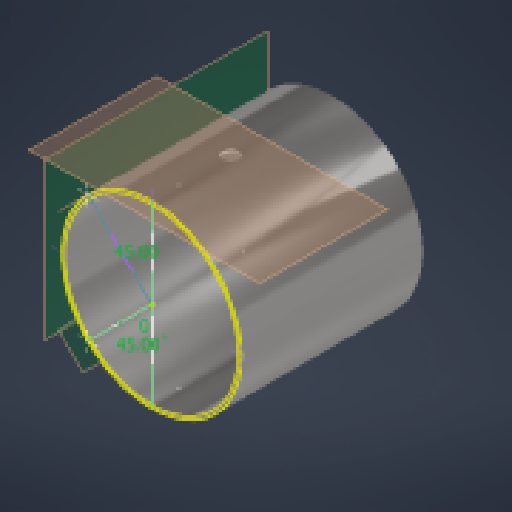
# Autodesk Inventor part: Electromagnetic cover body
Saved by Autodesk Inventor 2026.3 (Build 303398000, 398)
## iProperties
Created: 2026-08-03
Part Number: Electromagnetic cover body
Material: Generic
Document SubType Name: Sheet Metal
Designer: matot
Density: 1 g/cm^3
Sheet Metal Rule: Default_mm
Appearance: Default
Author: matot
Autodesk Inventor part; units mm, degrees
ref_plane "YZ Plane" through (0, 0, 0) normal (1, 0, 0) x (0, 1, 0)
ref_plane "XZ Plane" through (0, 0, 0) normal (0, 1, 0) x (-1, 0, 0)
ref_plane "XY Plane" through (0, 0, 0) normal (0, 0, 1) x (1, 0, 0)
sketch "Sketch1" plane through (0, 0, 0) normal (0, 0, 1) x (1, 0, 0)
  circle A0 centre (0, 0) radius 57
  circle A1 centre (0, 0) radius 55
  dimension "d0" = 114
  dimension "d1" = 110
  constraints: 2 centre point, 2 coincident
  measures "d0" diameter of A0
  measures "d1" diameter of A1
extrude "Extrusion1" add sketch "Sketch1" along normal blind 115
sketch "Sketch2" plane through (0, 0, 115) normal (0, 0, 1) x (1, 0, 0)
  circle A0 centre (0, 0) radius 57 projected
  point P0 (0, 57)
  constraints: 1 vertical alignment, 1 other
ref_plane "Work Plane1" through (0, 57, 115) normal (0, 1, 0) x (-1, 0, 0)
sketch "Sketch3" plane through (0, 57, 115) normal (0, 1, 0) x (-1, 0, 0)
  line L0 (57, 0) -> (-57, 0) projected
  point P0 (0, -115)
  point P1 (0, -50)
  dimension "d4" = 50
  measures "d4" distance from line of L0 point (0, -50)
hole "Hole1" at (0, 57, 65) direction (0, -1, 0) diameter 10 depth 20 tip angle 118
sketch "Sketch4" plane through (0, 0, 115) normal (0, 0, 1) x (1, 0, 0)
  circle A0 centre (0, 0) radius 57 projected
  point P0 (-57, 0)
  point P1 (57, 0)
  constraints: 1 horizontal alignment, 1 other
ref_plane "Work Plane3" through (-57, 0, 115) normal (-1, 0, 0) x (0, -1, 0)
sketch "Sketch6" plane through (0, 0, 115) normal (0, 0, 1) x (1, 0, 0)
  circle A0 centre (0, 0) radius 57 projected
  point P0 (0, 57)
  constraints: 1 vertical alignment, 1 other
ref_plane "Work Plane4" through (0, 57, 115) normal (0, 1, 0) x (-1, 0, 0)
sketch "Sketch7" plane through (0, 57, 115) normal (0, 1, 0) x (-1, 0, 0)
  line L0 (57, 0) -> (-57, 0) projected
  point P0 (0, -115)
  point P1 (0, -17.607)
  dimension "d20" = 17.607
  measures "d20" distance from line of point (0, -17.607) L0
hole "Hole3" at (0, 57, 97.393) direction (0, -1, 0) diameter 2 end through all
sketch "Sketch8" plane through (0, 0, 115) normal (0, 0, 1) x (1, 0, 0)
  circle A0 centre (0, 0) radius 57 projected
  circle A1 centre (0, 0) radius 55 projected
  line L0 (-40.3051, -40.3051) -> (0, 0)
  line L1 (0, -57) -> (0, 0)
  line L2 (-40.3051, 40.3051) -> (0, -0.029)
  line L3 (0, -0.029) -> (0, 57)
  dimension "d28" = 45
  dimension "d29" = 45
  dimension "d30" = 0
  constraints: 8 end point, 4 point on circle, 2 vertical
  measures "d30" horizontal distance of point (0, 0) L2.end
ref_plane "Work Plane5" through (-40.3051, -40.3051, 115) normal (-0.7071068, -0.7071068, 0) x (0.7071068, -0.7071068, 0)
ref_plane "Work Plane6" through (-40.3051, 40.3051, 115) normal (-0.7071068, 0.7071068, 0) x (-0.7071068, -0.7071068, 0)
sketch "Sketch9" plane through (-40.3051, 40.3051, 115) normal (-0.7071068, 0.7071068, 0) x (-0.7071068, -0.7071068, 0)
  line L0 (57, 0) -> (-57, 0) projected
  point P0 (0, -115)
  point P1 (0, -17.607)
  dimension "d31" = 17.607
  measures "d31" distance from line of point (0, -17.607) L0
hole "Hole4" at (-40.3051, 40.3051, 97.393) direction (0.7071068, -0.7071068, 0) diameter 2 end through all
sketch "Sketch10" plane through (-40.3051, -40.3051, 115) normal (-0.7071068, -0.7071068, 0) x (0.7071068, -0.7071068, 0)
  line L0 (57, 0) -> (-57, 0) projected
  point P0 (0, -115)
  point P1 (0, -17.607)
  dimension "d39" = 17.607
  measures "d39" distance from line of L0 point (0, -17.607)
hole "Hole5" at (-40.3051, -40.3051, 97.393) direction (0.7071068, 0.7071068, 0) diameter 2 end through all
equation "\"d26\" = Thickness"
equation "\"BendRadius\" = Thickness"
equation "\"BendReliefWidth\" = Thickness"
equation "\"BendReliefDepth\" = 0.5 * Thickness"
equation "\"CornerReliefSize\" = 4 * Thickness"
equation "\"MinimumRemnant\" = 2 * Thickness"
equation "\"TransitionRadius\" = BendRadius"
equation "\"JacobiRadiusSize\" = BendRadius"
equation "\"GapSize\" = Thickness"
equation "\"Thickness\" = 0.5"
body "Solid1"
